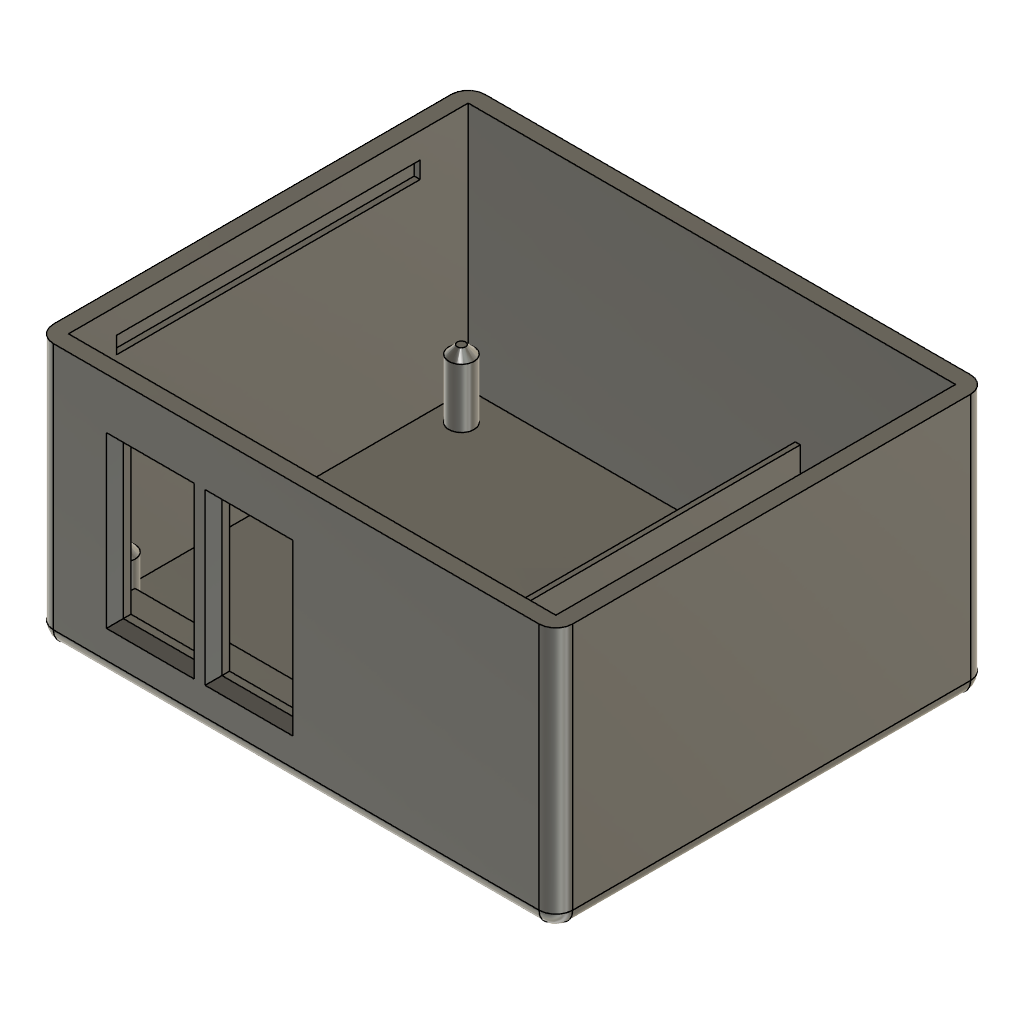
TURTLE_Case_BaseV3 (Autodesk Fusion 360 design; units mm, degrees)
Autodesk Fusion 360 part; units mm, degrees
(part 1 of 2)
sketch "Sketch1" plane through (0, 0, 0) normal (0, 0, 1) x (1, 0, 0)
  line L0 (19.1, 22.9) -> (-19.1, 22.9) construction
  line L1 (-19.1, 22.9) -> (-19.1, -22.9) construction
  line L2 (19.1, -22.9) -> (19.1, 22.9) construction
  line L3 (19.1, 22.9) -> (-19.1, -22.9) construction
  line L4 (-19.1, 22.9) -> (19.1, -22.9) construction
  line L5 (18.1, -21.701047) -> (18.1, -21.7) construction
  circle A0 centre (16.3, -20.1) radius 1.8 construction
  circle A1 centre (-16.3, -20.1) radius 1.8 construction
  line L6 (-7.845315, -9.406164) -> (-6.5, -9.406164) construction
  line L7 (-19.1, -22.9) -> (19.1, -22.9) construction
  line L8 (7.3, -22.9) -> (0.3, -22.9) construction
  line L9 (0.3, -22.9) -> (0.3, -10.480854) construction
  line L10 (0.3, -10.480854) -> (7.3, -10.480854) construction
  line L11 (7.3, -10.480854) -> (7.3, -22.9) construction
  line L12 (-11.4, -22.9) -> (-4.4, -22.9) construction
  line L13 (-4.4, -22.9) -> (-4.4, -10.450796) construction
  line L14 (-4.4, -10.450796) -> (-11.4, -10.450796) construction
  line L15 (-11.4, -10.450796) -> (-11.4, -22.9) construction
  line L16 (20.1, 22.9) -> (20.1, 23.7) construction
  line L17 (25.2, 25.2) -> (32.7, 25.2) construction
  line L18 (32.7, 25.2) -> (25.2, 25.2) construction
  line L19 (25.2, 25.2) -> (25.2, 16) construction
  line L20 (25.2, 16) -> (32.7, 16) construction
  line L21 (32.7, 16) -> (32.7, 25.2) construction
  line L22 (32.7, 25.2) -> (32.7, 23.7) construction
  line L23 (32.7, 23.7) -> (37.9, 23.7) construction
  line L24 (37.9, 23.7) -> (20.1, 23.7) construction
  line L25 (20.1, 23.7) -> (20.1, -19.5) construction
  line L26 (37.9, -19.5) -> (37.9, 23.7) construction
  line L27 (37.9, 23.7) -> (-19.1, 23.7) construction
  line L28 (-19.1, 23.7) -> (-19.1, -22.9) construction
  line L29 (-19.1, -22.9) -> (37.9, -22.9) construction
  line L30 (37.9, -22.9) -> (37.9, 23.7) construction
  line L31 (38.3, 24.1) -> (-19.5, 24.1) construction
  line L32 (-19.5, 24.1) -> (-19.5, -23.3) construction
  line L33 (-19.5, -23.3) -> (38.3, -23.3) construction
  line L34 (38.3, -23.3) -> (38.3, 24.1) construction
  line L35 (-19.5, 24.1) -> (38.3, 24.1)
  line L36 (38.3, 24.1) -> (38.3, -23.3)
  line L37 (38.3, -23.3) -> (-19.5, -23.3)
  line L38 (-19.5, -23.3) -> (-19.5, 24.1)
  line L39 (19.1, 22.9) -> (19.3, 22.9) construction
  line L40 (20.1, 22.9) -> (19.9, 22.9) construction
  line L41 (19.9, 23.699999) -> (19.9, -23.3)
  line L42 (19.9, -23.3) -> (19.3, -23.3)
  line L43 (19.3, -23.3) -> (19.3, 23.699999)
  line L44 (19.3, 23.699999) -> (19.3, 24.1)
  line L45 (19.9, 23.699999) -> (19.9, 24.1)
  circle A2 centre (-16.3, -20.1) radius 1.5
  circle A3 centre (16.3, -20.1) radius 1.5
  line L46 (25.2, 25.2) -> (25.2, 16) construction
  line L47 (16.764629, 20.1) -> (16.797966, 20.1) construction
  circle A4 centre (16.653553, 20.453553) radius 1.5
  circle A5 centre (-16.512132, 20.312132) radius 1.5
  arc A6 (-17.572792, 21.372792) -> (-17.704058, 21.226331) centre (-16.3, 20.1) ccw construction
  line L48 (38.3, -19.9) -> (38.3, -19.4) construction
  line L49 (-14.93946, -20.1) -> (-14.93946, -20.6)
  line L50 (-14.93946, -20.1) -> (14.949771, -20.1)
  line L51 (14.949771, -20.1) -> (14.949771, -23.3)
  line L52 (14.949771, -23.3) -> (-14.93946, -23.3)
  line L53 (-14.93946, -23.3) -> (-14.93946, -20.1)
  line L54 (-14.93946, -20.6) -> (-14.570838, -20.6)
  line L55 (14.949771, -20.6) -> (14.950326, -20.6)
  line L56 (40.2, -25.2) -> (-21.4, -25.2)
  line L57 (-21.4, -25.2) -> (-21.4, 26)
  line L58 (-21.4, 26) -> (40.2, 26)
  line L59 (40.2, 26) -> (40.2, -25.2)
  line L60 (41.2, -26.2) -> (-22.4, -26.2)
  line L61 (-22.4, -26.2) -> (-22.4, 27)
  line L62 (-22.4, 27) -> (41.2, 27)
  line L63 (41.2, 27) -> (41.2, -26.2)
  line L64 (32.7, 24.072882) -> (25.2, 24.072882)
  line L65 (25.2, 24.072882) -> (25.2, 18.072882)
  line L66 (25.2, 18.072882) -> (32.7, 18.072882)
  line L67 (32.7, 18.072882) -> (32.7, 24.072882)
  line L68 (38.3, -19.65) -> (19.9, -19.65)
  line L69 (20.1, -19.498913) -> (19.9, -19.5)
  dimension "d1" = 38.2
  dimension "d2" = 45.8
  dimension "d5" = 3.6
  dimension "d7" = 2.8
  dimension "d13" = 7
  dimension "d14" = 11.8
  dimension "d15" = 7
  dimension "d16" = 7.7
  dimension "d17" = 1
  dimension "d23" = 7.5
  dimension "d24" = 9.2
  dimension "d25" = 1.5
  dimension "d26" = 5.2
  dimension "d27" = 17.8
  dimension "d28" = 43.2
  dimension "d31" = 0.4
  dimension "d36" = 0.2
  dimension "d37" = 0.2
  dimension "d54" = 3
  dimension "d57" = 3
  dimension "d67" = 3
  dimension "d69" = 0.3
  dimension "d70" = 3
  dimension "d89" = 0.5
  dimension "d237" = -1
  dimension "d283" = 6
  constraint horizontal L0
  constraint perpendicular L0 L1
  constraint parallel L1 L2
  constraint coincident L3 origin
  constraint coincident L4 origin
  constraint horizontal L6
  constraint perpendicular L2 L7
  constraint horizontal L8
  constraint vertical L9
  constraint horizontal L10
  constraint vertical L11
  constraint coincident L7 L8.start
  constraint horizontal L12
  constraint vertical L13
  constraint horizontal L14
  constraint vertical L15
  constraint coincident L7 L12.start
  constraint perpendicular L16 L17
  constraint horizontal L18
  constraint vertical L19
  constraint horizontal L20
  constraint vertical L21
  constraint perpendicular L17 L22
  constraint perpendicular L22 L23
  constraint horizontal L24
  constraint vertical L25
  constraint vertical L26
  constraint horizontal L27
  constraint vertical L28
  constraint horizontal L29
  constraint vertical L30
  constraint horizontal L35
  constraint vertical L36
  constraint horizontal L37
  constraint vertical L38
  constraint perpendicular L2 L39
  constraint perpendicular L16 L40
  constraint vertical L41
  constraint horizontal L42
  constraint vertical L43
  constraint coincident L37 L41.end
  constraint coincident L35 L44.end
  constraint perpendicular L35 L44
  constraint coincident L31 L45.end
  constraint perpendicular L31 L45
  constraint concentric A0 A3
  constraint perpendicular L24 L46
  constraint coincident L34 L48.start
  constraint horizontal L47
  constraint coincident L41 L69.end
  constraint perpendicular L49 L54
  constraint horizontal L50
  constraint vertical L51
  constraint horizontal L52
  constraint vertical L53
  constraint collinear L54 L55
  constraint horizontal L64
  constraint vertical L65
  constraint horizontal L66
  constraint vertical L67
  constraint midpoint L48 L68.start
  constraint coincident L41 L68.end
  constraint perpendicular L41 L68
  measures "d1" distance of L1.end L2.start
  measures "d2" distance of L0.end L1.end
  measures "d5" diameter of A0
  measures "d7" distance of L2 A0.centre
  measures "d13" distance of L8.start L8.end
  measures "d14" distance of L2 L11
  measures "d15" distance of L12.start L12.end
  measures "d16" distance of L1 L15
  measures "d17" distance of L0.start L16.start
  measures "d23" distance of L17.end L17.start
  measures "d24" distance of L17.end L20.end
  measures "d25" distance of L17.end L22.end
  measures "d26" distance of L22.end L23.end
  measures "d27" distance of L23.end L16.end
  measures "d28" distance of L23.end L26.start
  measures "d36" distance of L0.start L39.end
  measures "d37" distance of L16.start L40.end
  measures "d54" diameter of A2
  measures "d57" diameter of A3
  measures "d67" diameter of A4
  measures "d70" diameter of A5
  measures "d89" distance of L48.start L48.end
extrude "Extrude1" add sketch "Sketch1" along normal blind 2 contours L35 L37 L38 L43 L44 A2 A3 L50 L51 L53 | L35 L37 L41 L42 L43 L44 L45 | L35 L36 L41 L45 L68 | L64 L65 L66 L67 picked at (5.168729, 6.497646) picked at (19.5, -6.366667) picked at (30.3, -7.025706) picked at (30.2, 20.072882) makes body 1
extrude "Extrude2" add sketch "Sketch1" along normal blind 10.2 contours L36 L37 L41 L68 | L56 L57 L58 L59 picked at (32.166667, -22.083333) picked at (11.249924, -24.566667) bodies 1
extrude "Extrude16" add sketch "Sketch1" along normal blind 6 contours L37 A2 A3 L50 L51 L52 L53 picked at (4.93994, -22.289549) bodies 1
extrude "Extrude3" add sketch "Sketch1" along normal blind 10 contours A2 L53 L54 | A2 L49 L50 L53 | A3 L50 L51 | A3 L50 L51 | A2 L49 L50 L53 L54 | A4 | A5 picked at (-14.909178, -20.61481) picked at (-16.841416, -20.032888) picked at (16.844339, -20.025479) picked at (14.853094, -20.156215) picked at (-14.905751, -20.378979) picked at (17.036708, 19.891568) picked at (-16.878658, 19.67729) bodies 1
extrude "Extrude12" add sketch "Sketch1" along normal blind 16 contours L35 L37 L41 L42 L43 L44 L45 picked at (19.5, -6.366667) bodies 1
extrude "Extrude32" add sketch "Sketch1" along normal blind 6 contours L64 L65 L66 L67 picked at (30.2, 20.072882) bodies 1
ref_plane "WorkPlane1" through (9.4, 0.4, 10.2) normal (0, 0, 1) x (1, 0, 0)
sketch "Sketch3" plane through (0, 0, 10.2) normal (0, 0, 1) x (1, 0, 0)
  line L0 (25.2, 25.2) -> (25.2, 16)
  line L1 (32.7, 25.2) -> (25.2, 25.2)
  line L2 (32.7, 16) -> (32.7, 25.2)
  line L3 (25.2, 16) -> (32.7, 16)
  line L4 (25.199999, 24.099999) -> (24.899999, 24.099999) construction
  line L5 (32.699999, 24.099999) -> (32.999999, 24.099999) construction
  line L6 (24.899999, 24.099999) -> (32.999999, 24.099999)
  line L7 (32.999999, 24.099999) -> (32.999999, 25.999999)
  line L8 (24.899999, 25.999999) -> (24.899999, 24.099999)
  line L9 (0.3, -22.9) -> (0.3, -10.480854)
  line L10 (0.3, -10.480854) -> (7.3, -10.480854)
  line L11 (7.3, -10.480854) -> (7.3, -22.9)
  line L12 (-19.1, -22.9) -> (37.9, -22.9)
  line L13 (-4.4, -22.9) -> (-4.4, -10.450796)
  line L14 (-4.4, -10.450796) -> (-11.4, -10.450796)
  line L15 (-11.4, -10.450796) -> (-11.4, -22.9)
  line L16 (7.3, -22.9) -> (8, -22.9) construction
  line L17 (0.3, -22.9) -> (-0.4, -22.9) construction
  line L18 (-4.4, -22.9) -> (-3.7, -22.9) construction
  line L19 (8, -23.3) -> (8, -22.9)
  line L20 (-12.1, -22.9) -> (-12.1, -25.199999)
  line L21 (-3.7, -25.199999) -> (-3.7, -23.3)
  line L22 (-19.5, -23.3) -> (-19.5, 24.1)
  line L23 (-19.5, 24.1) -> (38.3, 24.1)
  line L24 (19.9, 23.699999) -> (19.9, -23.3)
  line L25 (19.3, -23.3) -> (19.3, 23.699999)
  line L26 (19.9, 23.699999) -> (19.9, 24.1)
  line L27 (19.3, 23.699999) -> (19.3, 24.1)
  line L28 (38.3, -23.3) -> (38.3, 24.1)
  line L29 (-19.5, -23.3) -> (38.3, -23.3)
  line L30 (19.9, -22.9) -> (38.3, -22.9)
  line L31 (38.3, -22.9) -> (38.3, -19.9)
  line L32 (19.9, -19.9) -> (19.9, -22.9)
  line L33 (38.3, 24.1) -> (38.3, -19.65)
  line L34 (19.9, -23.3) -> (19.3, -23.3)
  line L35 (24.899999, 24.099999) -> (33, 24.099999)
  line L36 (33, 24.099999) -> (33, 27)
  line L37 (33, 27) -> (24.899999, 27)
  line L38 (24.899999, 27) -> (24.899999, 24.099999)
  line L39 (-11.4, -22.9) -> (-3.691525, -22.9)
  line L40 (-3.691525, -26.2) -> (-12.1, -26.2)
  line L41 (-0.4, -22.9) -> (8.002335, -22.9)
  line L42 (8.002335, -23.3) -> (8.002335, -26.2)
  line L43 (8.002335, -26.2) -> (-0.4, -26.2)
  line L44 (-0.4, -26.2) -> (-0.4, -22.9)
  line L45 (-3.691525, -22.9) -> (-3.691525, -23.3)
  line L46 (-3.691525, -25.2) -> (-3.691525, -26.2)
  line L47 (-12.1, -26.2) -> (-12.1, -25.199999)
  line L48 (-3.7, -22.9) -> (-4.4, -22.9)
  line L49 (-11.4, -22.9) -> (-12.1, -22.9)
  line L50 (8, -22.9) -> (7.3, -22.9)
  line L51 (0.3, -22.9) -> (-0.4, -22.9)
  line L52 (-3.691525, -22.9) -> (-12.1, -22.9)
  line L53 (-12.1, -22.9) -> (-12.1, -26.2)
  line L54 (-12.1, -26.2) -> (-3.691525, -26.2)
  line L55 (-3.691525, -26.2) -> (-3.691525, -22.9)
  line L56 (19.3, -23.3) -> (-19.5, -23.3)
  line L57 (-19.5, -23.3) -> (-19.5, 24.1)
  line L58 (-19.5, 24.1) -> (19.3, 24.1)
  line L59 (19.3, 24.1) -> (19.9, 24.1)
  line L60 (40.2, 26) -> (-21.4, 26)
  line L61 (-21.4, 26) -> (-21.4, -25.2)
  line L62 (-21.4, -25.2) -> (40.2, -25.2)
  line L63 (40.2, -25.2) -> (40.2, 26)
  line L64 (38.3, -19.65) -> (19.9, -19.65)
  line L65 (19.9, -19.65) -> (19.9, -23.3)
  line L66 (19.9, 24.1) -> (38.3, 24.1)
  dimension "d59" = 0.3
  dimension "d60" = 0.3
  dimension "d71" = 0.7
  dimension "d72" = 0.7
  dimension "d73" = 0.7
  constraint perpendicular L0 L4
  constraint perpendicular L2 L5
  constraint perpendicular L6 L7
  constraint parallel L7 L8
  constraint perpendicular L2 L6
  constraint coincident L11.end L16.start
  constraint perpendicular L11 L16
  constraint coincident L9.start L17.start
  constraint perpendicular L9 L17
  constraint coincident L13.start L18.start
  constraint perpendicular L13 L18
  constraint horizontal L50
  constraint vertical L19
  constraint horizontal L48
  constraint vertical L20
  constraint vertical L21
  constraint horizontal L30
  constraint vertical L31
  constraint vertical L32
  constraint coincident L24 L30.start
  constraint coincident L12 L30.start
  constraint horizontal L35
  constraint vertical L36
  constraint horizontal L37
  constraint vertical L38
  constraint horizontal L39
  constraint vertical L45
  constraint horizontal L40
  constraint vertical L47
  constraint horizontal L41
  constraint vertical L42
  constraint horizontal L43
  constraint vertical L44
  constraint coincident L29 L21.end
  constraint collinear L45 L46
  constraint collinear L48 L49
  constraint collinear L50 L51
  constraint coincident L29 L19.start
  constraint horizontal L52
  constraint vertical L53
  constraint horizontal L54
  constraint vertical L55
  measures "d71" distance of L11.end L16.end
  measures "d72" distance of L9.start L17.end
  measures "d73" distance of L13.start L18.end
extrude "Extrude5" cut sketch "Sketch3" against normal blind 3.9 contours L0 L1 L2 L6 L23 L35 L66 | L0 L1 L2 L6 L7 L8 L23 L35 L36 L38 L60 L66 | L36 L37 L38 L60 | L40 L46 L47 L53 L54 L55 L62 | L20 L21 L29 L53 L56 L62 | L29 L42 L44 L56 L62 | L42 L43 L44 L62 | L12 L20 L29 L39 L45 L48 L49 L52 L53 L55 L56 | L21 L29 L55 L56 L62 | L12 L19 L29 L41 L44 L50 L51 L56 picked at (27.7, 24.833333) picked at (27.7, 25.733333) picked at (30.3, 26.666667) picked at (-6.497175, -25.866667) picked at (-9.3, -23.933333) picked at (5.200778, -24.566667) picked at (2.400778, -25.533333) picked at (-6.733333, -23.166667) picked at (-3.69435, -24.566666) picked at (2.633333, -23.166667) bodies 1
extrude "Extrude13" add sketch "Sketch3" along normal blind 14.2 contours L0 L1 L2 L6 L23 L35 L66 | L0 L1 L2 L6 L7 L8 L23 L35 L36 L38 L60 L66 | L8 L20 L22 L23 L29 L38 L53 L56 L57 L58 L59 L60 L61 L62 L66 | L7 L23 L28 L29 L31 L33 L34 L36 L42 L56 L60 L62 L63 L66 | L29 L44 L55 L56 L62 picked at (27.7, 24.833333) picked at (27.7, 25.733333) picked at (7.6, 25.366666) picked at (39.566667, -6.283333) picked at (-2.59435, -24.566667) bodies 1
sketch "Sketch10" plane through (0, 0, 24.4) normal (0, 0, 1) x (-1, 0, 0)
  line L0 (19.5, -24.1) -> (-38.3, -24.1)
  line L1 (3.691525, 23.3) -> (12.1, 23.3)
  line L2 (12.1, 23.3) -> (12.1, 25.2)
  line L3 (3.691525, 25.2) -> (3.691525, 23.3)
  line L4 (0.4, 25.2) -> (0.4, 23.3)
  line L5 (0.4, 23.3) -> (3.691525, 23.3)
  line L6 (3.691525, 23.3) -> (3.691525, 25.2)
  line L7 (-8.002335, 23.3) -> (0.4, 23.3)
  line L8 (0.4, 23.3) -> (0.4, 25.2)
  line L9 (-8.002335, 25.2) -> (-8.002335, 23.3)
  line L10 (12.1, 23.3) -> (19.5, 23.3)
  line L11 (19.5, 23.3) -> (19.5, -24.1)
  line L12 (-38.3, -24.1) -> (-38.3, 23.3)
  line L13 (-38.3, 23.3) -> (-8.002335, 23.3)
  line L14 (-8.002335, 23.3) -> (-8.002335, 25.2)
  line L15 (-8.002335, 25.2) -> (-40.2, 25.2)
  line L16 (-40.2, 25.2) -> (-40.2, -26)
  line L17 (-40.2, -26) -> (21.4, -26)
  line L18 (21.4, -26) -> (21.4, 25.2)
  line L19 (21.4, 25.2) -> (12.1, 25.2)
  line L20 (12.1, 25.2) -> (12.1, 23.3)
  line L21 (12.1, 25.2) -> (3.691525, 25.2)
  line L22 (3.691525, 25.2) -> (0.4, 25.2)
  line L23 (0.4, 25.2) -> (-8.002335, 25.2)
extrude "Extrude22" add sketch "Sketch10" along normal blind 7 contours L0 L2 L9 L10 L11 L12 L13 L14 L15 L16 L17 L18 L19 L20 | L1 L2 L3 L6 L20 L21 | L4 L7 L8 L9 L14 L23 | L3 L4 L5 L6 L8 L22 picked at (0.233333, -25.366667) picked at (6.49435, 24.566667) picked at (-5.201557, 24.566667) picked at (2.59435, 23.933333) bodies 1
sketch "Sketch13" plane through (0, 0, 31.4) normal (0, 0, 1) x (-1, 0, 0)
  line L0 (-38.3, 23.3) -> (19.5, 23.3)
  line L1 (-7.925814, 23.3) -> (-7.925814, 23.1) construction
  line L2 (-38.3, 23.3) -> (-38.3, -0.4) construction
  line L3 (19.5, 23.3) -> (19.5, -0.4) construction
  line L4 (-38.3, -0.4) -> (-38.3, 17.6) construction
  line L5 (-38.3, -0.4) -> (-38.3, -18.4) construction
  line L6 (19.5, -0.4) -> (19.5, 17.6) construction
  line L7 (19.5, -0.4) -> (19.5, -18.4) construction
  line L8 (19.5, 17.6) -> (18.5, 17.6) construction
  line L9 (19.5, 17.6) -> (18.5, 17.6)
  line L10 (19.5, -18.4) -> (19.3, -18.4)
  line L11 (19.3, -18.4) -> (18.3, -18.4)
  line L12 (18.3, -18.4) -> (19.3, -18.4)
  line L13 (19.3, 17.6) -> (18.3, 17.6)
  line L14 (19.5, 23.3) -> (19.5, -24.1)
  line L15 (19.5, -24.1) -> (-38.3, -24.1)
  line L16 (-38.3, -24.1) -> (-38.3, 23.3)
  line L17 (21.4, 25.2) -> (-40.2, 25.2)
  line L18 (-40.2, 25.2) -> (-40.2, -26)
  line L19 (-40.2, -26) -> (21.4, -26)
  line L20 (21.4, -26) -> (21.4, 25.2)
  line L21 (-37.1, 10.6) -> (-38.1, 10.6) construction
  line L22 (-37.1, -16.4) -> (-37.1, 10.6)
  line L23 (-37.1, 10.6) -> (-38.1, 10.6)
  line L24 (-38.1, 10.6) -> (-38.1, -16.4)
  line L25 (-38.1, -16.4) -> (-37.1, -16.4)
  line L26 (-38.1, -16.4) -> (-38.299999, -16.4)
  line L27 (-38.299999, -16.4) -> (-38.299999, 10.6)
  line L28 (-38.299999, 10.6) -> (-38.1, 10.6)
  line L29 (19.3, -18.4) -> (19.5, -18.4)
  line L30 (19.5, -18.4) -> (19.5, 17.6)
  line L31 (19.5, 17.6) -> (19.3, 17.6)
  line L32 (19.3, 17.6) -> (19.3, -18.4)
  line L33 (18.3, 17.6) -> (18.3, -18.4)
  line L34 (19.3, 17.6) -> (19.3, -18.4)
  line L35 (-38.1, -16.4) -> (-38.1, 10.6)
  line L36 (18.3, -22.9) -> (-37.1, -22.9)
  line L37 (-37.1, 22.1) -> (18.3, 22.1)
  line L38 (18.3, 17.6) -> (18.3, -18.4)
  line L39 (19.3, 17.6) -> (19.3, -18.4)
  line L40 (-37.1, -16.4) -> (-37.1, 10.6)
  line L41 (-38.1, -16.4) -> (-38.1, 10.6)
  line L42 (18.3, 22.1) -> (19.5, 22.1)
  line L43 (-37.1, 22.1) -> (-38.299999, 22.1)
  line L44 (18.3, -22.9) -> (19.5, -22.9)
  line L45 (-37.1, -22.9) -> (-38.299999, -22.9)
  dimension "d189" = 0.2
  dimension "d192" = 23.7
  dimension "d193" = 23.7
  dimension "d194" = 18
  dimension "d195" = 18
  dimension "d196" = 18
  dimension "d197" = 18
  dimension "d199" = 1
  constraint coincident L0.start L2.start
  constraint perpendicular L0 L2
  constraint coincident L0.end L3.start
  constraint perpendicular L0 L3
  constraint parallel L2 L4
  constraint parallel L3 L6
  constraint perpendicular L3 L8
  constraint perpendicular L7 L10
  constraint perpendicular L7 L11
  constraint parallel L12 L13
  constraint perpendicular L22 L23
  constraint parallel L22 L24
  constraint parallel L23 L25
  constraint perpendicular L21 L22
  constraint horizontal L26
  constraint vertical L27
  constraint horizontal L28
  constraint horizontal L29
  constraint vertical L30
  constraint horizontal L31
  constraint vertical L32
  constraint coincident L3 L42.end
  constraint coincident L14 L44.end
  constraint perpendicular L14 L44
  constraint perpendicular L16 L45
  measures "d192" distance of L0.start L2.end
  measures "d193" distance of L0.end L3.end
  measures "d194" distance of L2.end L4.end
  measures "d195" distance of L2.end L5.end
  measures "d196" distance of L3.end L6.end
  measures "d197" distance of L3.end L7.end
  measures "d199" distance of L6.end L8.end
extrude "Extrude23" add sketch "Sketch13" along normal blind 5 separate body contours L0 L14 L16 L37 L42 L43 | L9 L10 L11 L12 L13 L14 L16 L22 L23 L25 L26 L28 L29 L31 L33 L36 L37 L38 L40 L42 L43 L44 L45 | L16 L24 L26 L27 L28 L35 L41 | L9 L10 L14 L29 L30 L31 L32 L34 L39 | L22 L23 L24 L25 L35 L40 L41 | L9 L11 L12 L13 L32 L33 L34 L38 L39 | L14 L15 L16 L36 L44 L45 | L17 L18 L19 L20 picked at (-18.633333, 22.9) picked at (-0.166667, 3.266667) picked at (-38.166667, 1.6) picked at (19.366667, -6.4) picked at (-37.766667, -7.4) picked at (18.7, -6.4) picked at (-18.633333, -23.7) picked at (-39.566667, -5.733333) makes body 2
extrude "Extrude25" add sketch "Sketch13" against normal blind 5 contours L22 L23 L24 L25 L35 L40 L41 | L9 L11 L12 L13 L32 L33 L34 L38 L39 picked at (-37.766667, -7.4) picked at (18.7, -6.4) bodies 2
ref_plane "WorkPlane2" through (9.4, 0.4, 33.9) normal (1, 0, 0) x (0, 1, 0)
sketch "Sketch19" plane through (38.1, 0, 0) normal (1, 0, 0) x (0, 1, 0)
  line L0 (-10.6, 26.4) -> (16.4, 26.4)
  line L1 (16.4, 26.4) -> (-10.6, 26.4)
  line L2 (-10.6, 26.4) -> (-10.6, 28.4)
  line L3 (-10.6, 28.4) -> (16.4, 28.4)
  line L4 (16.4, 28.4) -> (16.4, 26.4)
  line L5 (16.4, 31.4) -> (-10.6, 31.4)
  line L6 (-10.6, 31.4) -> (-10.6, 26.4)
  line L7 (16.4, 26.4) -> (16.4, 31.4)
  dimension "d269" = 2
  constraint perpendicular L1 L2
  constraint parallel L1 L3
  constraint parallel L2 L4
  constraint coincident L0.start L1.end
  constraint coincident L0.end L1.start
  measures "d269" distance of L0.end L3.end
sketch "Sketch26" plane through (-19.3, 0, 0) normal (-1, 0, 0) x (0, -1, 0)
  line L0 (17.6, 31.4) -> (-18.4, 31.4)
  line L1 (-18.4, 31.4) -> (-18.4, 26.4)
  line L2 (-18.4, 26.4) -> (17.6, 26.4)
  line L3 (17.6, 26.4) -> (17.6, 31.4)
  line L4 (17.6, 26.4) -> (-18.402292, 26.4)
  line L5 (-18.402292, 26.4) -> (-18.402292, 28.4)
  line L6 (-18.402292, 28.4) -> (17.6, 28.4)
  line L7 (17.6, 28.4) -> (17.6, 26.4)
  dimension "d327" = 2
  constraint horizontal L4
  constraint vertical L5
  constraint horizontal L6
  constraint vertical L7
  constraint coincident L2.end L3.start
  measures "d327" distance of L2.end L6.end
extrude "Extrude27" add sketch "Sketch26" along normal blind 0.7 contours L1 L2 L3 L4 L6 L7 picked at (-6.4, 27.733333) bodies 2
extrude "Extrude31" add sketch "Sketch19" along normal blind 0.7 contours L0 L1 L2 L3 L4 L6 L7 picked at (-1.6, 27.733333) bodies 2
sketch "Sketch18" plane through (40.2, 0, 0) normal (1, 0, 0) x (0, 1, 0)
  line L0 (-25.2, 31.4) -> (26, 31.4)
  line L1 (26, 31.4) -> (26, 36.4)
  line L2 (26, 36.4) -> (-25.2, 36.4)
  line L3 (-25.2, 36.4) -> (-25.2, 31.4)
  line L4 (-25.2, 31.4) -> (0.4, 31.4) construction
  line L5 (0.4, 31.4) -> (5.4, 31.4) construction
  line L6 (0.4, 31.4) -> (-4.6, 31.4) construction
  line L7 (-4.6, 31.4) -> (5.4, 31.4)
  line L8 (5.4, 31.4) -> (5.4, 33.9)
  line L9 (5.4, 33.9) -> (-4.6, 33.9)
  line L10 (-4.6, 33.9) -> (-4.6, 31.4)
  dimension "d257" = 25.6
  dimension "d258" = 5
  dimension "d259" = 5
  dimension "d260" = 10
  dimension "d261" = 2.5
  constraint coincident L0.start L3.end
  constraint perpendicular L3 L4
  constraint coincident L0 L5.end
  constraint parallel L4 L6
  constraint horizontal L7
  constraint vertical L8
  constraint horizontal L9
  constraint vertical L10
  measures "d257" distance of L0.start L4.end
  measures "d258" distance of L4.end L5.end
  measures "d259" distance of L4.end L6.end
  measures "d260" distance of L6.end L5.end
  measures "d261" distance of L6.end L9.end
extrude "Extrude30" cut sketch "Sketch18" against normal blind 1 contours L0 L7 L8 L9 L10 picked at (2.066667, 33.066667) bodies 2
mirror "Mirror2" about plane through (9.4, 0.4, 33.9) normal (1, 0, 0) of "Extrude30"
sketch "Sketch16" plane through (-19.5, 0, 0) normal (1, 0, 0) x (0, 1, 0)
  line L0 (-23.3, 2) -> (24.1, 2)
  line L1 (24.1, 2) -> (24.1, 31.4)
  line L2 (24.1, 31.4) -> (-23.3, 31.4)
  line L3 (-23.3, 31.4) -> (-23.3, 2)
  line L4 (-23.3, 31.4) -> (0.4, 31.4) construction
  line L5 (0.4, 31.4) -> (0.4, 28.4) construction
  line L6 (0.4, 28.4) -> (0.4, 26.4) construction
  line L7 (0.4, 26.4) -> (18.4, 26.4) construction
  line L8 (0.4, 26.4) -> (-17.6, 26.4) construction
  line L9 (-17.6, 26.4) -> (-17.6, 28.4) construction
  line L10 (-17.6, 28.4) -> (-17.6, 26.4)
  line L11 (-17.6, 26.4) -> (18.4, 26.4)
  line L12 (18.4, 26.4) -> (18.4, 28.4)
  line L13 (18.4, 28.4) -> (-17.6, 28.4)
  dimension "d222" = 23.7
  dimension "d223" = 3
  dimension "d224" = 2
  dimension "d225" = 18
  dimension "d226" = 18
  dimension "d227" = 2
  constraint coincident L2.end L3.start
  constraint midpoint L2 L4.end
  constraint perpendicular L4 L5
  constraint perpendicular L2 L6
  constraint perpendicular L6 L7
  constraint perpendicular L6 L8
  constraint perpendicular L8 L9
  constraint perpendicular L10 L11
  constraint parallel L10 L12
  constraint parallel L11 L13
  measures "d222" distance of L2.end L4.end
  measures "d223" distance of L4.end L5.end
  measures "d224" distance of L5.end L6.end
  measures "d225" distance of L6.end L7.end
  measures "d226" distance of L6.end L8.end
  measures "d227" distance of L8.end L9.end
extrude "Extrude28" cut sketch "Sketch16" against normal blind 0.7 contours L10 L11 L12 L13 picked at (6.4, 27.066667) bodies 1
extrude "Extrude29" cut sketch "Sketch13" along normal blind 3 contours L9 L10 L11 L12 L13 L14 L16 L22 L23 L25 L26 L28 L29 L31 L33 L36 L37 L38 L40 L42 L43 L44 L45 | L9 L10 L14 L29 L30 L31 L32 L34 L39 picked at (-0.166667, 3.266667) picked at (19.366667, -6.4) bodies 2
extrude "Extrude35" add sketch "Sketch13" against normal blind 2 contours L0 L14 L16 L37 L42 L43 | L14 L15 L16 L36 L44 L45 picked at (-18.633333, 22.9) picked at (-18.633333, -23.7) bodies 2
mirror "Mirror3" about plane through (9.4, 0.4, 33.9) normal (1, 0, 0) of "Extrude28"
sketch "Sketch17" plane through (9.4, 0, 0) normal (1, 0, 0) x (0, 1, 0)
fillet "Fillet16" radius 2 8 edges at (40.2, -25.2, 15.7) (40.2, 26, 15.7) (-21.4, 26, 15.7) (-21.4, -25.2, 15.7) (40.2, -25.2, 33.9) (40.2, 26, 33.9) (-21.4, 26, 33.9) (-21.4, -25.2, 33.9) on bodies 1 2
sketch "Sketch24" plane through (0, 0, 36.4) normal (0, 0, 1) x (-1, 0, 0)
  arc A0 (21.4, 23.2) -> (19.4, 25.2) centre (19.4, 23.2) ccw
  line L0 (19.4, 25.2) -> (-38.2, 25.2)
  arc A1 (-38.2, 25.2) -> (-40.2, 23.2) centre (-38.2, 23.2) ccw
  line L1 (-40.2, 23.2) -> (-40.2, -24)
  arc A2 (-40.2, -24) -> (-38.2, -26) centre (-38.2, -24) ccw
  line L2 (-38.2, -26) -> (19.4, -26)
  arc A3 (19.4, -26) -> (21.4, -24) centre (19.4, -24) ccw
  line L3 (21.4, -24) -> (21.4, 23.2)
  arc A4 (11.381116, -26) -> (21.4, -18.514137) centre (-2.785855, 3.408144) ccw
  arc A5 (11.066503, -23.794726) -> (16.139311, -20.512361) centre (4.942001, -8.768344) ccw
  arc A6 (16.139311, -20.512361) -> (21.4, -15.412687) centre (-2.563147, 4.04383) ccw
  arc A7 (21.4, -15.412687) -> (21.406161, -15.40482) centre (-2.734447, 3.496485) ccw
  arc A8 (8.860519, -25.530485) -> (10.472033, -26) centre (19.663325, 8.547571) ccw
  arc A9 (8.860519, -25.530485) -> (8.7, -26) centre (25.080489, -31.338018) ccw
  arc A10 (9.6, -23.399999) -> (10.224581, -23.754271) centre (15.292749, -14.091394) ccw
  arc A11 (9.534035, -23.0852) -> (9.6, -23.399999) centre (10.446701, -23.058267) ccw
  arc A12 (9.534035, -23.0852) -> (9.2, -14.6) centre (-44.113543, -20.94796) ccw
  arc A13 (6.7, -26) -> (7.630004, -23.54076) centre (-18.154084, -15.195524) ccw
  arc A14 (7.630004, -23.54076) -> (7.614071, -22.33379) centre (4.941798, -22.972657) ccw
  arc A15 (7.614071, -22.33379) -> (7.194843, -19.065179) centre (-155.48915, -41.592022) ccw
  arc A16 (7.194843, -19.065179) -> (7.05103, -15.289634) centre (-16.615008, -18.081596) ccw
  spline S0 degree 5 poles (7.05103, -15.289634) (7.055974, -15.268108) (7.063793, -15.226434) (7.069333, -15.168068) (7.064238, -15.098449) (7.033399, -15.021135) (6.964988, -14.939733) (6.843435, -14.836161) (6.663015, -14.698385) (6.437927, -14.528834) (6.193431, -14.338995) (5.95695, -14.143992) (5.74973, -13.957462) (5.577022, -13.785651) (5.42268, -13.623867) (5.260434, -13.461926) (5.062942, -13.288374) (4.811036, -13.094871) (4.504602, -12.881297) (4.159169, -12.654297) (3.799017, -12.424211) (3.451628, -12.202628) (3.141277, -11.99954) (2.883672, -11.820983) (2.678479, -11.665709) (2.508797, -11.525018) (2.350228, -11.386973) (2.177399, -11.23944) (1.971926, -11.07379) (1.728578, -10.88779) (1.451528, -10.684045) (1.151578, -10.468863) (0.842951, -10.250957) (0.540422, -10.040242) (0.255944, -9.846531) (-0.003148, -9.678504) (-0.234111, -9.543003) (-0.439412, -9.444175) (-0.626728, -9.382817) (-0.810094, -9.355286) (-1.006918, -9.353994) (-1.230608, -9.369399) (-1.485277, -9.391548) (-1.757498, -9.411864) (-2.022399, -9.424613) (-2.255372, -9.428554) (-2.440715, -9.42813) (-2.584413, -9.435774) (-2.715439, -9.470635) (-2.869624, -9.551888) (-3.075872, -9.692501) (-3.346173, -9.895104) (-3.680877, -10.155086) (-4.070917, -10.462277) (-4.501271, -10.803196) (-4.953843, -11.163039) (-5.41068, -11.527825) (-5.856841, -11.886339) (-6.283953, -12.232543) (-6.689365, -12.564822) (-7.074263, -12.884463) (-7.442143, -13.194408) (-7.797117, -13.497866) (-8.14235, -13.797047) (-8.478296, -14.091711) (-8.801357, -14.378104) (-9.101508, -14.646932) (-9.364342, -14.885476) (-9.575623, -15.082036) (-9.725377, -15.229965) (-9.811502, -15.331232) (-9.845232, -15.401729) (-9.850042, -15.470526) (-9.847164, -15.56717) (-9.846265, -15.713141) (-9.849947, -15.922764) (-9.857309, -16.203376) (-9.86728, -16.555871) (-9.878397, -16.97594) (-9.889083, -17.455233) (-9.897722, -17.982563) (-9.90282, -18.545066) (-9.903141, -19.129418) (-9.897831, -19.722945) (-9.886587, -20.314984) (-9.869662, -20.897257) (-9.847734, -21.463434) (-9.82181, -22.00892) (-9.79312, -22.530553) (-9.763015, -23.026347) (-9.732866, -23.495209) (-9.703953, -23.936672) (-9.677373, -24.350625) (-9.653917, -24.737023) (-9.634108, -25.095843) (-9.61826, -25.427087) (-9.608874, -25.670028) (-9.603708, -25.839835) (-9.601097, -25.94753) (-9.6, -26) knots 0 0 0 0 0 0 0.01052632 0.02105263 0.03157895 0.04210526 0.05263158 0.06315789 0.07368421 0.08421053 0.09473684 0.10526316 0.11578947 0.12631579 0.13684211 0.14736842 0.15789474 0.16842105 0.17894737 0.18947368 0.2 0.21052632 0.22105263 0.23157895 0.24210526 0.25263158 0.26315789 0.27368421 0.28421053 0.29473684 0.30526316 0.31578947 0.32631579 0.33684211 0.34736842 0.35789474 0.36842105 0.37894737 0.38947368 0.4 0.41052632 0.42105263 0.43157895 0.44210526 0.45263158 0.46315789 0.47368421 0.48421053 0.49473684 0.50526316 0.51578947 0.52631579 0.53684211 0.54736842 0.55789474 0.56842105 0.57894737 0.58947368 0.6 0.61052632 0.62105263 0.63157895 0.64210526 0.65263158 0.66315789 0.67368421 0.68421053 0.69473684 0.70526316 0.71578947 0.72631579 0.73684211 0.74736842 0.75789474 0.76842105 0.77894737 0.78947368 0.8 0.81052632 0.82105263 0.83157895 0.84210526 0.85263158 0.86315789 0.87368421 0.88421053 0.89473684 0.90526316 0.91578947 0.92631579 0.93684211 0.94736842 0.95789474 0.96842105 0.97894737 0.98947368 1 1 1 1 1 1
  spline S1 degree 5 poles (21.4, -10.5) (21.368142, -10.478327) (21.300204, -10.432697) (21.18563, -10.357394) (21.007513, -10.243267) (20.743623, -10.078213) (20.44167, -9.892281) (20.108177, -9.688583) (19.754073, -9.472349) (19.396053, -9.251561) (19.057107, -9.037267) (18.760563, -8.841494) (18.525096, -8.675477) (18.35874, -8.547627) (18.254689, -8.461913) (18.182941, -8.415311) (18.09497, -8.398156) (17.946327, -8.398728) (17.719741, -8.407572) (17.432766, -8.419545) (17.120947, -8.43203) (16.826725, -8.444009) (16.587054, -8.455056) (16.419081, -8.463722) (16.315761, -8.468458) (16.255305, -8.471391) (16.207036, -8.482158) (16.138762, -8.519686) (16.022237, -8.603792) (15.840458, -8.746511) (15.589361, -8.949122) (15.274065, -9.205734) (14.906597, -9.505048) (14.503066, -9.832826) (14.081014, -10.174102) (13.656862, -10.515359) (13.242927, -10.847068) (12.845915, -11.164919) (12.468512, -11.468281) (12.110302, -11.759266) (11.768961, -12.041547) (11.441297, -12.319308) (11.124399, -12.596105) (10.816656, -12.873836) (10.519009, -13.151487) (10.235572, -13.424528) (9.972452, -13.686211) (9.7369, -13.928513) (9.536324, -14.143229) (9.377379, -14.322979) (9.264985, -14.462299) (9.214185, -14.539315) (9.198415, -14.577331) (9.197819, -14.593905) (9.2, -14.6) knots 0 0 0 0 0 0 0.02 0.04 0.06 0.08 0.1 0.12 0.14 0.16 0.18 0.2 0.22 0.24 0.26 0.28 0.3 0.32 0.34 0.36 0.38 0.4 0.42 0.44 0.46 0.48 0.5 0.52 0.54 0.56 0.58 0.6 0.62 0.64 0.66 0.68 0.7 0.72 0.74 0.76 0.78 0.8 0.82 0.84 0.86 0.88 0.9 0.92 0.94 0.96 0.98 1 1 1 1 1 1
  arc A17 (10.224581, -23.754271) -> (11.066503, -23.794726) centre (10.689067, -22.868691) ccw
  spline S2 degree 5 poles (21.4, -7.9) (21.301553, -7.855402) (21.109573, -7.767271) (20.836348, -7.638265) (20.501546, -7.472642) (20.132094, -7.276525) (19.811263, -7.09212) (19.538134, -6.920997) (19.311111, -6.765796) (19.12775, -6.630398) (18.984566, -6.520388) (18.876884, -6.442707) (18.799122, -6.3979) (18.745046, -6.37328) (18.707992, -6.334984) (18.680099, -6.247929) (18.650588, -6.10436) (18.608169, -5.920746) (18.545051, -5.721498) (18.460838, -5.525993) (18.365412, -5.336662) (18.273751, -5.14634) (18.201521, -4.943446) (18.160654, -4.717672) (18.154199, -4.466298) (18.177879, -4.192958) (18.222974, -3.904881) (18.278822, -3.610586) (18.33527, -3.317572) (18.385665, -3.02954) (18.427165, -2.746086) (18.45943, -2.463927) (18.483809, -2.177645) (18.502334, -1.88063) (18.516772, -1.565943) (18.527728, -1.227185) (18.535004, -0.858934) (18.53787, -0.45722) (18.535362, -0.019987) (18.526571, 0.452457) (18.510948, 0.956923) (18.488562, 1.48698) (18.460477, 2.032214) (18.428692, 2.578929) (18.395731, 3.112033) (18.364344, 3.616575) (18.337148, 4.079442) (18.316307, 4.490959) (18.303184, 4.846592) (18.298016, 5.148487) (18.299549, 5.407396) (18.304793, 5.643527) (18.309748, 5.87997) (18.310024, 6.136776) (18.3015, 6.425014) (18.280957, 6.740283) (18.246772, 7.058016) (18.200017, 7.345499) (18.145601, 7.572669) (18.093254, 7.722962) (18.058929, 7.805114) (18.065137, 7.862051) (18.131097, 7.944043) (18.260449, 8.076961) (18.440977, 8.257351) (18.652649, 8.466336) (18.873294, 8.678053) (19.084953, 8.869908) (19.280724, 9.033201) (19.462761, 9.170829) (19.638863, 9.292846) (19.819631, 9.412871) (20.015257, 9.543984) (20.232857, 9.695325) (20.477195, 9.873015) (20.751086, 10.08068) (20.994957, 10.272233) (21.191987, 10.430456) (21.329616, 10.542407) (21.4, 10.6) knots 0 0 0 0 0 0 0.01333333 0.02666667 0.04 0.05333333 0.06666667 0.08 0.09333333 0.10666667 0.12 0.13333333 0.14666667 0.16 0.17333333 0.18666667 0.2 0.21333333 0.22666667 0.24 0.25333333 0.26666667 0.28 0.29333333 0.30666667 0.32 0.33333333 0.34666667 0.36 0.37333333 0.38666667 0.4 0.41333333 0.42666667 0.44 0.45333333 0.46666667 0.48 0.49333333 0.50666667 0.52 0.53333333 0.54666667 0.56 0.57333333 0.58666667 0.6 0.61333333 0.62666667 0.64 0.65333333 0.66666667 0.68 0.69333333 0.70666667 0.72 0.73333333 0.74666667 0.76 0.77333333 0.78666667 0.8 0.81333333 0.82666667 0.84 0.85333333 0.86666667 0.88 0.89333333 0.90666667 0.92 0.93333333 0.94666667 0.96 0.97333333 0.98666667 1 1 1 1 1 1
  spline S3 degree 5 poles (15.9, -4.9) (15.831672, -4.948807) (15.693229, -5.048124) (15.480198, -5.202207) (15.185409, -5.417884) (14.799605, -5.704188) (14.398495, -6.005949) (13.986236, -6.320536) (13.569977, -6.643376) (13.160491, -6.96754) (12.773434, -7.282912) (12.426012, -7.578383) (12.1329, -7.844551) (11.902111, -8.076442) (11.731485, -8.275826) (11.603252, -8.454812) (11.484774, -8.635307) (11.341496, -8.840309) (11.145949, -9.087809) (10.891057, -9.381884) (10.591354, -9.711646) (10.272529, -10.057791) (9.964199, -10.397031) (9.691394, -10.707363) (9.466625, -10.972947) (9.281489, -11.189271) (9.113956, -11.359714) (8.935876, -11.492028) (8.720042, -11.595026) (8.448213, -11.674872) (8.109983, -11.735262) (7.782322, -11.769562) (7.503862, -11.787718) (7.303706, -11.796466) (7.2, -11.8) knots 0 0 0 0 0 0 0.03333333 0.06666667 0.1 0.13333333 0.16666667 0.2 0.23333333 0.26666667 0.3 0.33333333 0.36666667 0.4 0.43333333 0.46666667 0.5 0.53333333 0.56666667 0.6 0.63333333 0.66666667 0.7 0.73333333 0.76666667 0.8 0.83333333 0.86666667 0.9 0.93333333 0.96666667 1 1 1 1 1 1
  spline S4 degree 5 poles (7.2, -11.8) (7.194221, -11.802855) (7.182122, -11.807523) (7.162346, -11.811398) (7.132729, -11.810312) (7.09053, -11.798733) (7.044005, -11.777628) (6.994569, -11.748272) (6.942933, -11.711978) (6.887871, -11.669619) (6.825427, -11.621253) (6.751066, -11.566606) (6.661229, -11.505381) (6.555583, -11.437748) (6.436671, -11.364229) (6.308238, -11.285297) (6.173973, -11.201058) (6.036057, -11.110892) (5.893853, -11.013136) (5.744828, -10.905566) (5.585405, -10.785863) (5.411858, -10.652086) (5.221149, -10.503126) (5.011883, -10.339224) (4.784944, -10.162291) (4.54283, -9.97539) (4.289186, -9.782343) (4.028257, -9.587292) (3.764377, -9.394276) (3.501452, -9.206807) (3.242423, -9.027437) (2.988786, -8.857356) (2.739958, -8.695877) (2.493802, -8.540882) (2.247374, -8.389466) (1.997583, -8.238493) (1.7419, -8.085208) (1.479019, -7.927803) (1.209604, -7.766047) (0.936865, -7.601781) (0.667551, -7.439771) (0.41121, -7.287045) (0.178317, -7.151233) (-0.021278, -7.039186) (-0.179995, -6.955532) (-0.294229, -6.901142) (-0.365802, -6.87188) (-0.40416, -6.856559) (-0.423134, -6.840599) (-0.436757, -6.810622) (-0.454996, -6.759262) (-0.484273, -6.683794) (-0.528631, -6.584035) (-0.590767, -6.460238) (-0.672491, -6.312508) (-0.774843, -6.140978) (-0.873628, -5.984776) (-0.957287, -5.856977) (-1.017312, -5.767047) (-1.048387, -5.7209) knots 0 0 0 0 0 0 0.01818182 0.03636364 0.05454545 0.07272727 0.09090909 0.10909091 0.12727273 0.14545455 0.16363636 0.18181818 0.2 0.21818182 0.23636364 0.25454545 0.27272727 0.29090909 0.30909091 0.32727273 0.34545455 0.36363636 0.38181818 0.4 0.41818182 0.43636364 0.45454545 0.47272727 0.49090909 0.50909091 0.52727273 0.54545455 0.56363636 0.58181818 0.6 0.61818182 0.63636364 0.65454545 0.67272727 0.69090909 0.70909091 0.72727273 0.74545455 0.76363636 0.78181818 0.8 0.81818182 0.83636364 0.85454545 0.87272727 0.89090909 0.90909091 0.92727273 0.94545455 0.96363636 0.98181818 1 1 1 1 1 1
  spline S5 degree 5 poles (-1.048387, -5.7209) (-1.055511, -5.715293) (-1.068602, -5.703979) (-1.084773, -5.68671) (-1.099372, -5.663086) (-1.106171, -5.632484) (-1.102276, -5.600616) (-1.089435, -5.567113) (-1.070812, -5.531372) (-1.050195, -5.492374) (-1.031196, -5.448484) (-1.016505, -5.397275) (-1.006992, -5.335276) (-1.002089, -5.258373) (-1.000361, -5.162318) (-0.999968, -5.043193) (-0.999194, -4.897963) (-0.996853, -4.724878) (-0.992138, -4.523089) (-0.984565, -4.2924) (-0.973877, -4.033007) (-0.962761, -3.802829) (-0.952978, -3.617611) (-0.945816, -3.48856) (-0.942075, -3.422642) knots 0 0 0 0 0 0 0.05 0.1 0.15 0.2 0.25 0.3 0.35 0.4 0.45 0.5 0.55 0.6 0.65 0.7 0.75 0.8 0.85 0.9 0.95 1 1 1 1 1 1
  spline S6 degree 5 poles (-0.942075, -3.422642) (-0.949476, -3.250059) (-0.964626, -2.908712) (-0.988397, -2.408147) (-1.022196, -1.763811) (-1.06792, -0.99763) (-1.116864, -0.271262) (-1.168365, 0.415631) (-1.2212, 1.064975) (-1.273307, 1.681466) (-1.321817, 2.272659) (-1.36355, 2.847324) (-1.395425, 3.414284) (-1.414867, 3.981252) (-1.420397, 4.553395) (-1.411498, 5.133475) (-1.39283, 5.604869) (-1.372434, 5.962648) (-1.356013, 6.203037) (-1.347097, 6.323698) knots 0 0 0 0 0 0 0.06666667 0.13333333 0.2 0.26666667 0.33333333 0.4 0.46666667 0.53333333 0.6 0.66666667 0.73333333 0.8 0.86666667 0.93333333 1 1 1 1 1 1
  spline S7 degree 5 poles (-1.347097, 6.323698) (-1.350434, 6.330747) (-1.355833, 6.345246) (-1.360113, 6.368201) (-1.358185, 6.401224) (-1.343312, 6.446813) (-1.31698, 6.497585) (-1.280731, 6.555175) (-1.235473, 6.621828) (-1.180244, 6.700385) (-1.111853, 6.79403) (-1.026526, 6.905594) (-0.921006, 7.037008) (-0.794079, 7.188586) (-0.647287, 7.358711) (-0.483968, 7.544417) (-0.308611, 7.741799) (-0.126101, 7.946481) (0.059015, 8.154076) (0.243212, 8.360611) (0.424837, 8.56305) (0.603901, 8.759267) (0.781589, 8.947882) (0.959867, 9.128146) (1.141051, 9.299807) (1.327387, 9.462981) (1.520642, 9.61803) (1.721654, 9.765423) (1.930524, 9.905788) (2.14688, 10.039983) (2.370103, 10.169154) (2.599582, 10.29481) (2.834933, 10.418876) (3.076274, 10.543777) (3.324382, 10.672456) (3.580237, 10.807924) (3.844644, 10.952882) (4.117811, 11.109306) (4.398963, 11.278055) (4.685906, 11.458447) (4.974679, 11.647897) (5.259009, 11.841396) (5.530324, 12.031474) (5.779411, 12.209645) (5.997826, 12.367615) (6.179328, 12.498544) (6.321468, 12.598371) (6.426748, 12.666922) (6.504864, 12.709587) (6.57153, 12.737195) (6.640237, 12.762173) (6.715646, 12.795501) (6.785992, 12.843349) (6.83483, 12.907181) (6.851568, 12.983971) (6.845181, 13.066052) (6.839049, 13.143086) (6.861119, 13.204413) (6.934031, 13.241718) (7.072097, 13.249681) (7.284065, 13.225086) (7.516111, 13.178126) (7.725898, 13.127337) (7.881638, 13.086561) (7.963478, 13.064444) knots 0 0 0 0 0 0 0.01666667 0.03333333 0.05 0.06666667 0.08333333 0.1 0.11666667 0.13333333 0.15 0.16666667 0.18333333 0.2 0.21666667 0.23333333 0.25 0.26666667 0.28333333 0.3 0.31666667 0.33333333 0.35 0.36666667 0.38333333 0.4 0.41666667 0.43333333 0.45 0.46666667 0.48333333 0.5 0.51666667 0.53333333 0.55 0.56666667 0.58333333 0.6 0.61666667 0.63333333 0.65 0.66666667 0.68333333 0.7 0.71666667 0.73333333 0.75 0.76666667 0.78333333 0.8 0.81666667 0.83333333 0.85 0.86666667 0.88333333 0.9 0.91666667 0.93333333 0.95 0.96666667 0.98333333 1 1 1 1 1 1
  spline S8 degree 5 poles (7.963478, 13.064444) (7.995566, 13.056054) (8.061021, 13.036743) (8.163038, 13.000181) (8.306745, 12.936217) (8.499053, 12.831197) (8.703486, 12.702305) (8.918868, 12.552099) (9.143045, 12.385178) (9.373642, 12.207161) (9.608976, 12.023401) (9.848959, 11.837733) (10.095905, 11.651345) (10.355703, 11.46122) (10.636409, 11.261438) (10.9462, 11.045166) (11.291611, 10.806345) (11.675502, 10.541633) (12.095408, 10.251988) (12.540948, 9.945117) (12.994838, 9.634567) (13.436345, 9.336539) (13.844034, 9.067359) (14.198707, 8.840771) (14.486472, 8.665084) (14.701342, 8.540808) (14.849241, 8.456868) (14.947314, 8.391528) (15.016738, 8.319809) (15.07736, 8.21907) (15.141189, 8.075802) (15.199526, 7.921993) (15.248244, 7.783697) (15.282923, 7.681324) (15.300814, 7.627593) knots 0 0 0 0 0 0 0.03333333 0.06666667 0.1 0.13333333 0.16666667 0.2 0.23333333 0.26666667 0.3 0.33333333 0.36666667 0.4 0.43333333 0.46666667 0.5 0.53333333 0.56666667 0.6 0.63333333 0.66666667 0.7 0.73333333 0.76666667 0.8 0.83333333 0.86666667 0.9 0.93333333 0.96666667 1 1 1 1 1 1
  spline S9 degree 5 poles (15.300814, 7.627593) (15.299143, 7.627499) (15.296974, 7.622492) (15.297231, 7.600517) (15.304601, 7.542296) (15.324716, 7.426331) (15.353173, 7.283017) (15.384998, 7.142894) (15.414738, 7.036344) (15.437928, 6.982565) (15.453224, 6.972551) (15.462179, 6.973715) (15.467041, 6.953013) (15.469413, 6.891406) (15.470551, 6.779224) (15.471579, 6.612768) (15.473599, 6.39177) (15.477598, 6.119122) (15.4844, 5.800008) (15.494603, 5.441282) (15.508524, 5.050776) (15.526122, 4.636585) (15.547033, 4.206642) (15.570667, 3.768465) (15.596285, 3.32885) (15.623085, 2.893578) (15.65028, 2.467121) (15.677184, 2.052337) (15.70329, 1.650177) (15.728358, 1.259344) (15.752483, 0.876079) (15.775981, 0.495095) (15.79929, 0.110387) (15.82287, -0.28391) (15.847099, -0.69268) (15.872178, -1.118984) (15.898024, -1.563196) (15.924172, -2.022175) (15.949663, -2.488312) (15.973156, -2.950537) (15.993061, -3.39547) (16.00766, -3.808509) (16.015233, -4.174936) (16.014183, -4.481017) (16.003162, -4.715115) (15.981195, -4.868789) (15.95449, -4.924124) (15.929265, -4.927051) (15.910139, -4.911872) (15.9, -4.9) knots 0 0 0 0 0 0 0.02222222 0.04444444 0.06666667 0.08888889 0.11111111 0.13333333 0.15555556 0.17777778 0.2 0.22222222 0.24444444 0.26666667 0.28888889 0.31111111 0.33333333 0.35555556 0.37777778 0.4 0.42222222 0.44444444 0.46666667 0.48888889 0.51111111 0.53333333 0.55555556 0.57777778 0.6 0.62222222 0.64444444 0.66666667 0.68888889 0.71111111 0.73333333 0.75555556 0.77777778 0.8 0.82222222 0.84444444 0.86666667 0.88888889 0.91111111 0.93333333 0.95555556 0.97777778 1 1 1 1 1 1
  spline S10 degree 5 poles (21.4, 14.1) (21.368296, 14.081135) (21.297986, 14.038561) (21.171815, 13.960173) (20.962163, 13.826588) (20.632425, 13.611861) (20.239297, 13.351596) (19.791379, 13.050256) (19.303262, 12.715408) (18.796595, 12.358342) (18.302632, 11.995257) (17.859837, 11.646579) (17.503646, 11.333424) (17.258434, 11.074778) (17.127852, 10.884287) (17.087506, 10.767435) (17.072604, 10.718011) (16.979648, 10.716451) (16.737395, 10.737398) (16.369686, 10.756128) (15.957934, 10.752757) (15.600332, 10.71645) (15.374012, 10.649233) (15.292243, 10.570952) (15.273869, 10.521141) (15.217326, 10.536589) (15.078994, 10.626406) (14.864927, 10.778092) (14.603733, 10.969882) (14.322942, 11.182455) (14.034494, 11.405648) (13.741584, 11.634736) (13.440275, 11.869248) (13.123311, 12.110691) (12.782785, 12.360903) (12.413776, 12.619756) (12.015198, 12.884981) (11.58934, 13.153011) (11.141817, 13.419504) (10.681335, 13.679999) (10.219593, 13.930537) (9.771007, 14.168233) (9.352814, 14.392019) (8.984047, 14.602842) (8.681306, 14.802232) (8.455292, 14.991298) (8.306651, 15.169305) (8.222983, 15.332999) (8.173058, 15.474132) (8.118946, 15.588407) (8.031347, 15.686065) (7.906046, 15.804206) (7.757697, 15.995428) (7.609515, 16.312219) (7.484765, 16.793435) (7.396675, 17.448397) (7.349475, 18.260946) (7.340622, 19.195723) (7.362594, 20.203637) (7.404865, 21.227651) (7.455794, 22.20842) (7.504541, 23.08997) (7.542994, 23.825415) (7.567645, 24.382538) (7.5816, 24.749753) (7.596296, 24.941219) (7.634032, 25.0043) (7.721883, 25.002706) (7.882942, 24.992277) (8.131919, 25.008568) (8.47776, 25.073418) (8.835373, 25.17266) (9.149743, 25.275349) (9.37983, 25.356357) (9.5, 25.399999) knots 0 0 0 0 0 0 0.01428571 0.02857143 0.04285714 0.05714286 0.07142857 0.08571429 0.1 0.11428571 0.12857143 0.14285714 0.15714286 0.17142857 0.18571429 0.2 0.21428571 0.22857143 0.24285714 0.25714286 0.27142857 0.28571429 0.3 0.31428571 0.32857143 0.34285714 0.35714286 0.37142857 0.38571429 0.4 0.41428571 0.42857143 0.44285714 0.45714286 0.47142857 0.48571429 0.5 0.51428571 0.52857143 0.54285714 0.55714286 0.57142857 0.58571429 0.6 0.61428571 0.62857143 0.64285714 0.65714286 0.67142857 0.68571429 0.7 0.71428571 0.72857143 0.74285714 0.75714286 0.77142857 0.78571429 0.8 0.81428571 0.82857143 0.84285714 0.85714286 0.87142857 0.88571429 0.9 0.91428571 0.92857143 0.94285714 0.95714286 0.97142857 0.98571429 1 1 1 1 1 1
  spline S11 degree 5 poles (9.5, 25.399999) (9.56817, 25.388971) (9.707528, 25.3621) (9.925616, 25.307348) (10.234548, 25.205384) (10.650011, 25.030468) (11.091427, 24.811307) (11.551706, 24.554955) (12.018623, 24.273787) (12.478552, 23.981817) (12.920455, 23.690788) (13.339359, 23.406749) (13.741129, 23.125409) (14.143469, 22.831093) (14.569062, 22.503259) (15.040124, 22.121639) (15.572954, 21.671412) (16.17107, 21.1497) (16.824315, 20.56643) (17.513397, 19.94006) (18.212809, 19.294846) (18.894256, 18.657616) (19.529953, 18.054688) (20.095655, 17.509025) (20.574654, 17.036499) (20.957984, 16.645697) (21.184942, 16.401515) (21.309992, 16.257239) (21.373335, 16.178283) (21.4, 16.143112) knots 0 0 0 0 0 0 0.04 0.08 0.12 0.16 0.2 0.24 0.28 0.32 0.36 0.4 0.44 0.48 0.52 0.56 0.6 0.64 0.68 0.72 0.76 0.8 0.84 0.88 0.92 0.96 1 1 1 1 1 1
  spline S12 degree 5 poles (5.128885, 15.849289) (4.813949, 15.647129) (4.115918, 15.195359) (3.104434, 14.527087) (1.89738, 13.698387) (0.658888, 12.788092) (-0.326481, 11.98684) (-1.018754, 11.334209) (-1.448689, 10.824927) (-1.662995, 10.450713) (-1.728715, 10.199506) (-1.734563, 10.054957) (-1.799856, 9.995258) (-2.056931, 9.994059) (-2.536306, 10.026707) (-3.131376, 10.074417) (-3.691863, 10.127298) (-4.085859, 10.186885) (-4.286133, 10.270361) (-4.411759, 10.409878) (-4.622978, 10.635436) (-5.018246, 10.956378) (-5.614575, 11.360396) (-6.378614, 11.822512) (-7.24104, 12.310747) (-8.118357, 12.793375) (-8.930133, 13.244956) (-9.62141, 13.654202) (-10.171688, 14.026551) (-10.583526, 14.378464) (-10.875722, 14.733605) (-11.075078, 15.118421) (-11.207919, 15.557664) (-11.294633, 16.071026) (-11.351539, 16.672592) (-11.39122, 17.369604) (-11.423418, 18.161664) (-11.455793, 19.039272) (-11.494306, 19.984305) (-11.542905, 20.972906) (-11.603394, 21.977762) (-11.675222, 22.970614) (-11.755304, 23.924652) (-11.837802, 24.816997) (-11.913955, 25.631066) (-11.971794, 26.359241) (-11.997496, 27.000849) (-11.976815, 27.559883) (-11.896552, 28.042766) (-11.74586, 28.456259) (-11.517994, 28.80492) (-11.27144, 29.033795) (-11.049937, 29.177689) (-10.88602, 29.261284) (-10.8, 29.299999) knots 0.00445908 0.00445908 0.00445908 0.00445908 0.00445908 0.00445908 0.02 0.04 0.06 0.08 0.1 0.12 0.14 0.16 0.18 0.2 0.22 0.24 0.26 0.28 0.3 0.32 0.34 0.36 0.38 0.4 0.42 0.44 0.46 0.48 0.5 0.52 0.54 0.56 0.58 0.6 0.62 0.64 0.66 0.68 0.7 0.72 0.74 0.76 0.78 0.8 0.82 0.84 0.86 0.88 0.9 0.92 0.94 0.96 0.98 1 1 1 1 1 1
  line L4 (-38.2, -26) -> (19.4, -26)
  line L5 (21.4, -24) -> (21.4, 23.2)
  arc A18 (19.4, -26) -> (21.4, -24) centre (19.4, -24) ccw
  arc A19 (21.4, 23.2) -> (19.4, 25.2) centre (19.4, 23.2) ccw
  line L6 (19.4, 25.2) -> (-38.2, 25.2)
  arc A20 (-38.2, 25.2) -> (-40.2, 23.2) centre (-38.2, 23.2) ccw
  line L7 (-40.2, 23.2) -> (-40.2, -24)
  arc A21 (-40.2, -24) -> (-38.2, -26) centre (-38.2, -24) ccw
  spline S13 degree 5 poles (5.588692, 16.69083) (5.588692, 16.720467) (5.588692, 16.892459) (5.588692, 17.212396) (5.588692, 17.692497) (5.588692, 18.352771) (5.588692, 19.185824) (5.588692, 20.070565) (5.588692, 21.006881) (5.588692, 21.991161) (5.588692, 23.019043) (5.588692, 23.873031) (5.588692, 24.530154) (5.588692, 24.975506) (5.588692, 25.2) knots 0.07910214 0.07910214 0.07910214 0.07910214 0.07910214 0.07910214 0.1 0.2 0.3 0.4 0.5 0.6 0.7 0.8 0.9 1 1 1 1 1 1
  arc A22 (5.128885, 15.849289) -> (5.588692, 16.69083) centre (4.588692, 16.69083) ccw